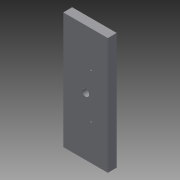
# Autodesk Inventor part: predni_komatex(0)
Saved by Autodesk Inventor 2015 (Build 190159000, 159)
## iProperties
Created: 2015-01-01
Part Number: predni_komatex(0)
Material: Generic
Document SubType Name: Modeling
Designer: Turboslimak
Density: 1 g/cm^3
Appearance: Default
Author: Turboslimak
Autodesk Inventor part; units mm, degrees
ref_plane "YZ Plane" through (0, 0, 0) normal (1, 0, 0) x (0, 1, 0)
ref_plane "XZ Plane" through (0, 0, 0) normal (0, 1, 0) x (-1, 0, 0)
ref_plane "XY Plane" through (0, 0, 0) normal (0, 0, 1) x (1, 0, 0)
sketch "Sketch1" plane through (0, 0, 0) normal (0, 1, 0) x (-1, 0, 0)
  line L0 (25, -65.5) -> (-25, -65.5)
  line L1 (-25, -65.5) -> (-25, 65.5)
  line L2 (-25, 65.5) -> (25, 65.5)
  line L3 (25, 65.5) -> (25, -65.5)
  circle A0 centre (0, 0) radius 4
  circle A1 centre (-6, -25) radius 1
  circle A2 centre (-6, 25) radius 1
  dimension "d0" = 50
  dimension "d1" = 131
  dimension "d4" = 8
  dimension "d10" = 2
  constraints: 8 end point, 3 centre point, 2 parallel, 1 coincident, 1 horizontal, 1 perpendicular
  measures "d0" distance of L1.end L2.end
  measures "d1" distance of L0.end L1.end
  measures "d4" diameter of A0
  measures "d10" diameter of A2
extrude "Extrusion1" add sketch "Sketch1" along normal blind 10 contours L0 L1 L2 L3 | A0 | A1 | A2
extrude "Extrusion2" cut sketch "Sketch1" along normal blind 10 contours A0 | A1 | A2
sketch "Sketch2" plane through (-25, 0, -65.5) normal (-1, 0, 0) x (0, 0, 1)
  circle A0 centre (65.5, 5) radius 1.25
  point P0 (65.5, 0)
  dimension "d14" = 2.5
  constraints: 1 centre point
  measures "d14" diameter of A0
extrude "Extrusion3" cut sketch "Sketch2" against normal blind 10
body "Solid1"
